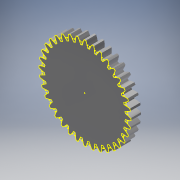
# Autodesk Inventor part: Цилиндрическое зубчатое зацепление2
Saved by Autodesk Inventor 2019 (Build 230136000, 136)
## iProperties
Created: 2020-02-27
Part Number: Цилиндрическое зубчатое зацепление2
Material: Steel
Document SubType Name: Modeling
Designer: Петров Иван
Categories: <?xml version="1.0" encoding="UTF-16"?> <MemberInstance><Categories><FamilyTemplate><FamilyTemplateParameter ValueType="xs:double" Id="1" ObjectReferenceKey="da_z" ObjectType="kUserParameterObject"/><FamilyTemplateParameter ValueType="xs:double" Id="2" ObjectReferenceKey="da_b" ObjectType="kUserParameterObject"/><FamilyTemplateParameter ValueType="xs:double" Id="3" ObjectReferenceKey="da_beta" ObjectType="kUserParameterObject"/><FamilyTemplateParameter ValueType="xs:double" Id="4" ObjectReferenceKey="da_da" ObjectType="kUserParameterObject"/><FamilyTemplateParameter ValueType="xs:double" Id="5" ObjectReferenceKey="da_aw" ObjectType="kUserParameterObject"/><FamilyTemplateParameter ValueType="xs:string" Id="6" ObjectReferenceKey="EAIAABAAAACIAQAAAAAAAIAAAAAAAAAA" ObjectType="83910656" SubObjectId="SurfaceGeometry"/></FamilyTemplate><ParamToTemplateMap><ParamToTemplate CategoryParameter="//CategoryParameter[@InternalName='046C89C9-8512-4d59-83FE-43B91F4F132A']" TemplateParameter="1"/><ParamToTemplate CategoryParameter="//CategoryParameter[@InternalName='2552DF32-E462-4b46-AEBF-C6C7768E72AC']" TemplateParameter="2"/><ParamToTemplate CategoryParameter="//CategoryParameter[@InternalName='C9EE641D-15FC-4fae-A226-E94C4372FDD7']" TemplateParameter="3"/><ParamToTemplate><ParamToTemplate CategoryParameter="//CategoryParameter[@InternalName='00B6519A-459B-49c7-AD84-2E56D39A5744']" ConstantValue="-1.183741"/></ParamToTemplate><ParamToTemplate><ParamToTemplate CategoryParameter="//CategoryParameter[@InternalName='04B31F0E-C7A6-4894-AA32-9629BEFACF47']" ConstantValue="1.000000"/></ParamToTemplate><ParamToTemplate><ParamToTemplate CategoryParameter="//CategoryParameter[@InternalName='43CBEC2E-7847-49e7-A936-2F7889FCB2D9']" ConstantValue="0.250000"/></ParamToTemplate><ParamToTemplate><ParamToTemplate CategoryParameter="//CategoryParameter[@InternalName='B1EFC894-105D-4ebd-86BF-FA20ED196853']" ConstantValue="0.350000"/></ParamToTemplate><ParamToTemplate><ParamToTemplate CategoryParameter="//CategoryParameter[@InternalName='51175063-3D10-4879-93E8-6246FE8B403D']" ConstantValue="2060000000.000000"/></ParamToTemplate><ParamToTemplate><ParamToTemplate CategoryParameter="//CategoryParameter[@InternalName='A3A52E27-4454-46a9-B0BD-C932399B70AF']" ConstantValue="0.300000"/></ParamToTemplate><ParamToTemplate><ParamToTemplate CategoryParameter="//CategoryParameter[@InternalName='91B76062-C214-41d9-B1B9-14D2AB99603D']" ConstantValue="0.175000"/></ParamToTemplate><ParamToTemplate><ParamToTemplate CategoryParameter="//CategoryParameter[@InternalName='374E806E-8B8A-4dda-A9AA-1039D6500AD2']" ConstantValue="5.714286"/></ParamToTemplate><ParamToTemplate><ParamToTemplate CategoryParameter="//CategoryParameter[@InternalName='2D373A89-B862-43d6-8D0B-0CBF12AB9F6C']" ConstantValue="0.523599"/></ParamToTemplate><ParamToTemplate CategoryParameter="//CategoryParameter[@InternalName='37777632-D6A2-4fac-9D53-DB8ACD95C989']" TemplateParameter="4"/><ParamToTemplate CategoryParameter="//CategoryParameter[@InternalName='FD1017F1-B727-4f7e-9707-0F86F1FF9423']" TemplateParameter="5"/><ParamToTemplate><ParamToTemplate CategoryParameter="//CategoryParameter[@InternalName='9E1B4470-B2D3-4ff1-B813-535BB4CDF51A']" ConstantValue="3520000.000000"/></ParamToTemplate><ParamToTemplate><ParamToTemplate CategoryParameter="//CategoryParameter[@InternalName='F8452263-BFF6-458c-9FB1-07C4B99E95CD']" ConstantValue="11400000.000000"/></ParamToTemplate><ParamToTemplate><ParamToTemplate CategoryParameter="//CategoryParameter[@InternalName='3E3BB259-FD49-497f-8171-6EBC954A3479']" ConstantValue="2.000000"/></ParamToTemplate><ParamToTemplate CategoryParameter="//CategoryParameter[@InternalName='27C3BAF2-7550-4e4b-AE2C-0DB134B7D9B7']" TemplateParameter="6"/></ParamToTemplateMap><Category DisplayName="Gear" InternalName="DC85795E-93AB-48d5-8EEE-5A27447B64BD" Mnemonic="Gear"><CategoryParameter DisplayName="z" InternalName="046C89C9-8512-4d59-83FE-43B91F4F132A" Mnemonic="z"/><CategoryParameter DisplayName="b" InternalName="2552DF32-E462-4b46-AEBF-C6C7768E72AC" Mnemonic="b"/><CategoryParameter DisplayName="||b|" InternalName="C9EE641D-15FC-4fae-A226-E94C4372FDD7" Mnemonic="beta"/><CategoryParameter DisplayName="x" InternalName="00B6519A-459B-49c7-AD84-2E56D39A5744" Mnemonic="x"/><CategoryParameter DisplayName="a*" InternalName="04B31F0E-C7A6-4894-AA32-9629BEFACF47" Mnemonic="a"/><CategoryParameter DisplayName="c*" InternalName="43CBEC2E-7847-49e7-A936-2F7889FCB2D9" Mnemonic="c"/><CategoryParameter DisplayName="r|.f|*" InternalName="B1EFC894-105D-4ebd-86BF-FA20ED196853" Mnemonic="rf"/><CategoryParameter DisplayName="E" InternalName="51175063-3D10-4879-93E8-6246FE8B403D" Mnemonic="E"/><CategoryParameter DisplayName="||m|" InternalName="A3A52E27-4454-46a9-B0BD-C932399B70AF" Mnemonic="mi"/><Category DisplayName="SpurGear" InternalName="26C5A22E-A91E-4dfd-A3B3-23CCAFAE1764" Mnemonic="SpurGear"><CategoryParameter DisplayName="m" InternalName="91B76062-C214-41d9-B1B9-14D2AB99603D" Mnemonic="m"/><CategoryParameter DisplayName="P" InternalName="374E806E-8B8A-4dda-A9AA-1039D6500AD2" Mnemonic="PP"/><CategoryParameter DisplayName="||a|" InternalName="2D373A89-B862-43d6-8D0B-0CBF12AB9F6C" Mnemonic="alpha"/><CategoryParameter DisplayName="d|.a|" InternalName="37777632-D6A2-4fac-9D53-DB8ACD95C989" Mnemonic="da"/><CategoryParameter DisplayName="a|.w|" InternalName="FD1017F1-B727-4f7e-9707-0F86F1FF9423" Mnemonic="aw"/><CategoryParameter DisplayName="||s||.Flim|" InternalName="9E1B4470-B2D3-4ff1-B813-535BB4CDF51A" Mnemonic="sFlim"/><CategoryParameter DisplayName="||s||.Hlim|" InternalName="F8452263-BFF6-458c-9FB1-07C4B99E95CD" Mnemonic="sHlim"/><CategoryParameter DisplayName="тип" InternalName="3E3BB259-FD49-497f-8171-6EBC954A3479" Mnemonic="type"/><CategoryParameter DisplayName="PitchDiameter" InternalName="27C3BAF2-7550-4e4b-AE2C-0DB134B7D9B7" Mnemonic="IDS_PITCHDIAM"/></Category></Category></Categories></MemberInstance>
Density: 1 g/cm^3
Appearance: Steel
CustomPartVersion: 1
Author: Петров Иван
Autodesk Inventor part; units mm, degrees
ref_plane "YZ Plane" through (0, 0, 0) normal (1, 0, 0) x (0, 1, 0)
ref_plane "XZ Plane" through (0, 0, 0) normal (0, 1, 0) x (-1, 0, 0)
ref_plane "XY Plane" through (0, 0, 0) normal (0, 0, 1) x (1, 0, 0)
sketch "Sketch1" plane through (0, 0, 0) normal (0, 0, 1) x (1, 0, 0)
  circle A0 centre (0, 0) radius 31
  dimension "d0" = 62
  constraints: 1 centre point
  measures "d0" diameter of A0
extrude "Extrusion1" add sketch "Sketch1" along normal blind 7
ref_plane "Work Plane2" through (0, 0, 3.5) normal (0, 0, 1) x (1, 0, 0)
sketch "Sketch2" plane through (0, 0, 0) normal (0, 0, -1) x (-1, 0, 0)
  circle A0 centre (0, 0) radius 31 projected
  circle A1 centre (0, 0) radius 30
  dimension "d3" = 60
  constraints: 1 centre point, 1 coincident
  measures "d3" diameter of A1
surface extrude "Средний диаметр" sketch "Sketch2" against normal through all shown no curves A1
ref_plane "Work Plane8" through (0, 0, 0) normal (0.9961947, 0.0871557, 0) x (0, 0, 1)
ref_plane "Work Plane9" through (0, 0, 0) normal (1, 0, 0) x (0, 1, 0)
spur gear teeth "Цилиндрическое зубчатое зацепление" teeth 36 pitch diameter 63 tip diameter 62 root diameter 54.4819 face width 7 start plane through (0, 0, 0) normal (0, 0, -1) x (-1, 0, 0)
sketch "Эскиз3" plane through (0, 0, 7) normal (0, 0, 1) x (1, 0, 0)
  arc A0 (-6.0478, 30.4043) -> (-6.4748, 26.4603) centre (11.6354, 26.4948) ccw projected
  arc A1 (-6.4748, 26.4603) -> (-7.6228, 26.1527) centre (0, 0) ccw projected
  arc A2 (-7.6228, 26.1527) -> (-9.9646, 29.3548) centre (-23.3239, 17.1275) ccw projected
  arc A3 (-9.9646, 29.3548) -> (-11.2356, 28.8922) centre (0, 0) ccw projected
  arc A4 (-11.2356, 28.8922) -> (-10.9712, 24.934) centre (6.8578, 28.1127) ccw projected
  arc A5 (-10.9712, 24.934) -> (-12.0484, 24.4317) centre (0, 0) ccw projected
  arc A6 (-12.0484, 24.4317) -> (-14.9107, 27.1785) centre (-25.9437, 12.8171) ccw projected
  arc A7 (-14.9107, 27.1785) -> (-16.082, 26.5023) centre (0, 0) ccw projected
  arc A8 (-16.082, 26.5023) -> (-15.1343, 22.65) centre (1.8719, 28.8765) ccw projected
  arc A9 (-15.1343, 22.65) -> (-16.1078, 21.9683) centre (0, 0) ccw projected
  arc A10 (-16.1078, 21.9683) -> (-19.4036, 24.1764) centre (-27.7753, 8.1173) ccw projected
  arc A11 (-19.4036, 24.1764) -> (-20.4397, 23.307) centre (0, 0) ccw projected
  arc A12 (-20.4397, 23.307) -> (-18.8375, 19.6779) centre (-3.1709, 28.7628) ccw projected
  arc A13 (-18.8375, 19.6779) -> (-19.6779, 18.8375) centre (0, 0) ccw projected
  arc A14 (-19.6779, 18.8375) -> (-23.307, 20.4397) centre (-28.7628, 3.1709) ccw projected
  arc A15 (-23.307, 20.4397) -> (-24.1764, 19.4036) centre (0, 0) ccw projected
  arc A16 (-24.1764, 19.4036) -> (-21.9683, 16.1078) centre (-8.1173, 27.7753) ccw projected
  arc A17 (-21.9683, 16.1078) -> (-22.65, 15.1343) centre (0, 0) ccw projected
  arc A18 (-22.65, 15.1343) -> (-26.5023, 16.082) centre (-28.8765, -1.8719) ccw projected
  arc A19 (-26.5023, 16.082) -> (-27.1785, 14.9107) centre (0, 0) ccw projected
  arc A20 (-27.1785, 14.9107) -> (-24.4317, 12.0484) centre (-12.8171, 25.9437) ccw projected
  arc A21 (-24.4317, 12.0484) -> (-24.934, 10.9712) centre (0, 0) ccw projected
  arc A22 (-24.934, 10.9712) -> (-28.8922, 11.2356) centre (-28.1127, -6.8578) ccw projected
  arc A23 (-28.8922, 11.2356) -> (-29.3548, 9.9646) centre (0, 0) ccw projected
  arc A24 (-29.3548, 9.9646) -> (-26.1527, 7.6228) centre (-17.1275, 23.3239) ccw projected
  arc A25 (-26.1527, 7.6228) -> (-26.4603, 6.4748) centre (0, 0) ccw projected
  arc A26 (-26.4603, 6.4748) -> (-30.4043, 6.0478) centre (-26.4948, -11.6354) ccw projected
  arc A27 (-30.4043, 6.0478) -> (-30.6392, 4.7158) centre (0, 0) ccw projected
  arc A28 (-30.6392, 4.7158) -> (-27.079, 2.9656) centre (-20.9174, 19.9954) ccw projected
  arc A29 (-27.079, 2.9656) -> (-27.1826, 1.7816) centre (0, 0) ccw projected
  arc A30 (-27.1826, 1.7816) -> (-30.9926, 0.6763) centre (-24.0718, -16.0594) ccw projected
  arc A31 (-30.9926, 0.6763) -> (-30.9926, -0.6763) centre (0, 0) ccw projected
  arc A32 (-30.9926, -0.6763) -> (-27.1826, -1.7816) centre (-24.0718, 16.0594) ccw projected
  arc A33 (-27.1826, -1.7816) -> (-27.079, -2.9656) centre (0, 0) ccw projected
  arc A34 (-27.079, -2.9656) -> (-30.6392, -4.7158) centre (-20.9174, -19.9954) ccw projected
  arc A35 (-30.6392, -4.7158) -> (-30.4043, -6.0478) centre (0, 0) ccw projected
  arc A36 (-30.4043, -6.0478) -> (-26.4603, -6.4748) centre (-26.4948, 11.6354) ccw projected
  arc A37 (-26.4603, -6.4748) -> (-26.1527, -7.6228) centre (0, 0) ccw projected
  arc A38 (-26.1527, -7.6228) -> (-29.3548, -9.9646) centre (-17.1275, -23.3239) ccw projected
  arc A39 (-29.3548, -9.9646) -> (-28.8922, -11.2356) centre (0, 0) ccw projected
  arc A40 (-28.8922, -11.2356) -> (-24.934, -10.9712) centre (-28.1127, 6.8578) ccw projected
  arc A41 (-24.934, -10.9712) -> (-24.4317, -12.0484) centre (0, 0) ccw projected
  arc A42 (-24.4317, -12.0484) -> (-27.1785, -14.9107) centre (-12.8171, -25.9437) ccw projected
  arc A43 (-27.1785, -14.9107) -> (-26.5023, -16.082) centre (0, 0) ccw projected
  arc A44 (-26.5023, -16.082) -> (-22.65, -15.1343) centre (-28.8765, 1.8719) ccw projected
  arc A45 (-22.65, -15.1343) -> (-21.9683, -16.1078) centre (0, 0) ccw projected
  arc A46 (-21.9683, -16.1078) -> (-24.1764, -19.4036) centre (-8.1173, -27.7753) ccw projected
  arc A47 (-24.1764, -19.4036) -> (-23.307, -20.4397) centre (0, 0) ccw projected
  arc A48 (-23.307, -20.4397) -> (-19.6779, -18.8375) centre (-28.7628, -3.1709) ccw projected
  arc A49 (-19.6779, -18.8375) -> (-18.8375, -19.6779) centre (0, 0) ccw projected
  arc A50 (-18.8375, -19.6779) -> (-20.4397, -23.307) centre (-3.1709, -28.7628) ccw projected
  arc A51 (-20.4397, -23.307) -> (-19.4036, -24.1764) centre (0, 0) ccw projected
  arc A52 (-19.4036, -24.1764) -> (-16.1078, -21.9683) centre (-27.7753, -8.1173) ccw projected
  arc A53 (-16.1078, -21.9683) -> (-15.1343, -22.65) centre (0, 0) ccw projected
  arc A54 (-15.1343, -22.65) -> (-16.082, -26.5023) centre (1.8719, -28.8765) ccw projected
  arc A55 (-16.082, -26.5023) -> (-14.9107, -27.1785) centre (0, 0) ccw projected
  arc A56 (-14.9107, -27.1785) -> (-12.0484, -24.4317) centre (-25.9437, -12.8171) ccw projected
  arc A57 (-12.0484, -24.4317) -> (-10.9712, -24.934) centre (0, 0) ccw projected
  arc A58 (-10.9712, -24.934) -> (-11.2356, -28.8922) centre (6.8578, -28.1127) ccw projected
  arc A59 (-11.2356, -28.8922) -> (-9.9646, -29.3548) centre (0, 0) ccw projected
  arc A60 (-9.9646, -29.3548) -> (-7.6228, -26.1527) centre (-23.3239, -17.1275) ccw projected
  arc A61 (-7.6228, -26.1527) -> (-6.4748, -26.4603) centre (0, 0) ccw projected
  arc A62 (-6.4748, -26.4603) -> (-6.0478, -30.4043) centre (11.6354, -26.4948) ccw projected
  arc A63 (-6.0478, -30.4043) -> (-4.7158, -30.6392) centre (0, 0) ccw projected
  arc A64 (-4.7158, -30.6392) -> (-2.9656, -27.079) centre (-19.9954, -20.9174) ccw projected
  arc A65 (-2.9656, -27.079) -> (-1.7816, -27.1826) centre (0, 0) ccw projected
  arc A66 (-1.7816, -27.1826) -> (-0.6763, -30.9926) centre (16.0594, -24.0718) ccw projected
  arc A67 (-0.6763, -30.9926) -> (0.6763, -30.9926) centre (0, 0) ccw projected
  arc A68 (0.6763, -30.9926) -> (1.7816, -27.1826) centre (-16.0594, -24.0718) ccw projected
  arc A69 (1.7816, -27.1826) -> (2.9656, -27.079) centre (0, 0) ccw projected
  arc A70 (2.9656, -27.079) -> (4.7158, -30.6392) centre (19.9954, -20.9174) ccw projected
  arc A71 (4.7158, -30.6392) -> (6.0478, -30.4043) centre (0, 0) ccw projected
  arc A72 (6.0478, -30.4043) -> (6.4748, -26.4603) centre (-11.6354, -26.4948) ccw projected
  arc A73 (6.4748, -26.4603) -> (7.6228, -26.1527) centre (0, 0) ccw projected
  arc A74 (7.6228, -26.1527) -> (9.9646, -29.3548) centre (23.3239, -17.1275) ccw projected
  arc A75 (9.9646, -29.3548) -> (11.2356, -28.8922) centre (0, 0) ccw projected
  arc A76 (11.2356, -28.8922) -> (10.9712, -24.934) centre (-6.8578, -28.1127) ccw projected
  arc A77 (10.9712, -24.934) -> (12.0484, -24.4317) centre (0, 0) ccw projected
  arc A78 (12.0484, -24.4317) -> (14.9107, -27.1785) centre (25.9437, -12.8171) ccw projected
  arc A79 (14.9107, -27.1785) -> (16.082, -26.5023) centre (0, 0) ccw projected
  arc A80 (16.082, -26.5023) -> (15.1343, -22.65) centre (-1.8719, -28.8765) ccw projected
  arc A81 (15.1343, -22.65) -> (16.1078, -21.9683) centre (0, 0) ccw projected
  arc A82 (16.1078, -21.9683) -> (19.4036, -24.1764) centre (27.7753, -8.1173) ccw projected
  arc A83 (19.4036, -24.1764) -> (20.4397, -23.307) centre (0, 0) ccw projected
  arc A84 (20.4397, -23.307) -> (18.8375, -19.6779) centre (3.1709, -28.7628) ccw projected
  arc A85 (18.8375, -19.6779) -> (19.6779, -18.8375) centre (0, 0) ccw projected
  arc A86 (19.6779, -18.8375) -> (23.307, -20.4397) centre (28.7628, -3.1709) ccw projected
  arc A87 (23.307, -20.4397) -> (24.1764, -19.4036) centre (0, 0) ccw projected
  arc A88 (24.1764, -19.4036) -> (21.9683, -16.1078) centre (8.1173, -27.7753) ccw projected
  arc A89 (21.9683, -16.1078) -> (22.65, -15.1343) centre (0, 0) ccw projected
  arc A90 (22.65, -15.1343) -> (26.5023, -16.082) centre (28.8765, 1.8719) ccw projected
  arc A91 (26.5023, -16.082) -> (27.1785, -14.9107) centre (0, 0) ccw projected
  arc A92 (27.1785, -14.9107) -> (24.4317, -12.0484) centre (12.8171, -25.9437) ccw projected
  arc A93 (24.4317, -12.0484) -> (24.934, -10.9712) centre (0, 0) ccw projected
  arc A94 (24.934, -10.9712) -> (28.8922, -11.2356) centre (28.1127, 6.8578) ccw projected
  arc A95 (28.8922, -11.2356) -> (29.3548, -9.9646) centre (0, 0) ccw projected
  arc A96 (29.3548, -9.9646) -> (26.1527, -7.6228) centre (17.1275, -23.3239) ccw projected
  arc A97 (26.1527, -7.6228) -> (26.4603, -6.4748) centre (0, 0) ccw projected
  arc A98 (26.4603, -6.4748) -> (30.4043, -6.0478) centre (26.4948, 11.6354) ccw projected
  arc A99 (30.4043, -6.0478) -> (30.6392, -4.7158) centre (0, 0) ccw projected
  arc A100 (30.6392, -4.7158) -> (27.079, -2.9656) centre (20.9174, -19.9954) ccw projected
  arc A101 (27.079, -2.9656) -> (27.1826, -1.7816) centre (0, 0) ccw projected
  arc A102 (27.1826, -1.7816) -> (30.9926, -0.6763) centre (24.0718, 16.0594) ccw projected
  arc A103 (30.9926, -0.6763) -> (30.9926, 0.6763) centre (0, 0) ccw projected
  arc A104 (30.9926, 0.6763) -> (27.1826, 1.7816) centre (24.0718, -16.0594) ccw projected
  arc A105 (27.1826, 1.7816) -> (27.079, 2.9656) centre (0, 0) ccw projected
  arc A106 (27.079, 2.9656) -> (30.6392, 4.7158) centre (20.9174, 19.9954) ccw projected
  arc A107 (30.6392, 4.7158) -> (30.4043, 6.0478) centre (0, 0) ccw projected
  arc A108 (30.4043, 6.0478) -> (26.4603, 6.4748) centre (26.4948, -11.6354) ccw projected
  arc A109 (26.4603, 6.4748) -> (26.1527, 7.6228) centre (0, 0) ccw projected
  arc A110 (26.1527, 7.6228) -> (29.3548, 9.9646) centre (17.1275, 23.3239) ccw projected
  arc A111 (29.3548, 9.9646) -> (28.8922, 11.2356) centre (0, 0) ccw projected
  arc A112 (28.8922, 11.2356) -> (24.934, 10.9712) centre (28.1127, -6.8578) ccw projected
  arc A113 (24.934, 10.9712) -> (24.4317, 12.0484) centre (0, 0) ccw projected
  arc A114 (24.4317, 12.0484) -> (27.1785, 14.9107) centre (12.8171, 25.9437) ccw projected
  arc A115 (27.1785, 14.9107) -> (26.5023, 16.082) centre (0, 0) ccw projected
  arc A116 (26.5023, 16.082) -> (22.65, 15.1343) centre (28.8765, -1.8719) ccw projected
  arc A117 (22.65, 15.1343) -> (21.9683, 16.1078) centre (0, 0) ccw projected
  arc A118 (21.9683, 16.1078) -> (24.1764, 19.4036) centre (8.1173, 27.7753) ccw projected
  arc A119 (24.1764, 19.4036) -> (23.307, 20.4397) centre (0, 0) ccw projected
  arc A120 (23.307, 20.4397) -> (19.6779, 18.8375) centre (28.7628, 3.1709) ccw projected
  arc A121 (19.6779, 18.8375) -> (18.8375, 19.6779) centre (0, 0) ccw projected
  arc A122 (18.8375, 19.6779) -> (20.4397, 23.307) centre (3.1709, 28.7628) ccw projected
  arc A123 (20.4397, 23.307) -> (19.4036, 24.1764) centre (0, 0) ccw projected
  arc A124 (19.4036, 24.1764) -> (16.1078, 21.9683) centre (27.7753, 8.1173) ccw projected
  arc A125 (16.1078, 21.9683) -> (15.1343, 22.65) centre (0, 0) ccw projected
  arc A126 (15.1343, 22.65) -> (16.082, 26.5023) centre (-1.8719, 28.8765) ccw projected
  arc A127 (16.082, 26.5023) -> (14.9107, 27.1785) centre (0, 0) ccw projected
  arc A128 (14.9107, 27.1785) -> (12.0484, 24.4317) centre (25.9437, 12.8171) ccw projected
  arc A129 (12.0484, 24.4317) -> (10.9712, 24.934) centre (0, 0) ccw projected
  arc A130 (10.9712, 24.934) -> (11.2356, 28.8922) centre (-6.8578, 28.1127) ccw projected
  arc A131 (11.2356, 28.8922) -> (9.9646, 29.3548) centre (0, 0) ccw projected
  arc A132 (9.9646, 29.3548) -> (7.6228, 26.1527) centre (23.3239, 17.1275) ccw projected
  arc A133 (7.6228, 26.1527) -> (6.4748, 26.4603) centre (0, 0) ccw projected
  arc A134 (6.4748, 26.4603) -> (6.0478, 30.4043) centre (-11.6354, 26.4948) ccw projected
  arc A135 (6.0478, 30.4043) -> (4.7158, 30.6392) centre (0, 0) ccw projected
  arc A136 (4.7158, 30.6392) -> (2.9656, 27.079) centre (19.9954, 20.9174) ccw projected
  arc A137 (2.9656, 27.079) -> (1.7816, 27.1826) centre (0, 0) ccw projected
  arc A138 (1.7816, 27.1826) -> (0.6763, 30.9926) centre (-16.0594, 24.0718) ccw projected
  arc A139 (0.6763, 30.9926) -> (-0.6763, 30.9926) centre (0, 0) ccw projected
  arc A140 (-0.6763, 30.9926) -> (-1.7816, 27.1826) centre (16.0594, 24.0718) ccw projected
  arc A141 (-1.7816, 27.1826) -> (-2.9656, 27.079) centre (0, 0) ccw projected
  arc A142 (-2.9656, 27.079) -> (-4.7158, 30.6392) centre (-19.9954, 20.9174) ccw projected
  arc A143 (-4.7158, 30.6392) -> (-6.0478, 30.4043) centre (0, 0) ccw projected
equation "\"d0\" = da_da"
equation "\"d1\" = da_b"
equation "\"d3\" = da_dw"
equation "\"d16\" = da_aw"
equation "\"d43\" = da_aw"
equation "\"d46\" = da_aw"
equation "\"da_da\" = 62"
equation "\"da_b\" = 7"
equation "\"da_dw\" = 60"
equation "\"da_aw\" = 45"
body "Solid1"
body "Srf1"
